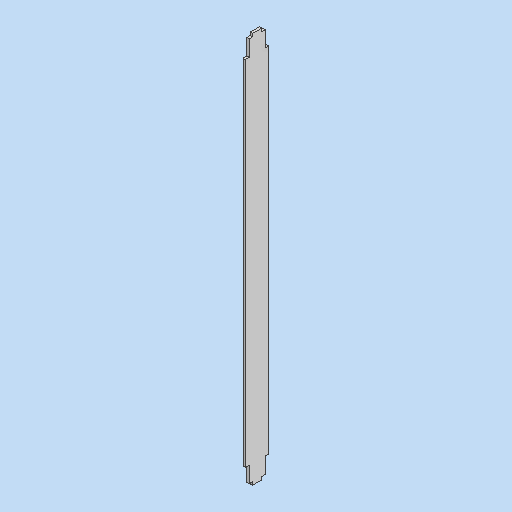
# Autodesk Inventor part: Acrly_Wand_1
Saved by Autodesk Inventor 2022 (Build 260153000, 153)
## iProperties
Created: 2021-12-15
Part Number: Acrly_Wand_1
Material: Generic
Document SubType Name: Modeling
Designer: Fabijansven
Density: 1 g/cm^3
Appearance: Default
Author: Fabijansven
Autodesk Inventor part; units mm, degrees
ref_plane "YZ Plane" through (0, 0, 0) normal (1, 0, 0) x (0, 1, 0)
ref_plane "XZ Plane" through (0, 0, 0) normal (0, 1, 0) x (-1, 0, 0)
ref_plane "XY Plane" through (0, 0, 0) normal (0, 0, 1) x (1, 0, 0)
sketch "Sketch1" plane through (0, 0, 0) normal (1, 0, 0) x (0, 1, 0)
  line L0 (0, 0) -> (822, 0)
  line L1 (822, 0) -> (822, -49.5)
  line L2 (822, -49.5) -> (0, -49.5)
  line L3 (0, -49.5) -> (0, 0)
  line L4 (822, 0) -> (815.75, 0)
  line L5 (815.75, 0) -> (815.75, -15)
  line L6 (815.75, -15) -> (822, -15)
  line L7 (822, -15) -> (822, 0)
  line L8 (822, 0) -> (782, 0)
  line L9 (782, 0) -> (782, -8)
  line L10 (782, -8) -> (822, -8)
  line L11 (822, -8) -> (822, 0)
  line L12 (856.5319, -24.75) -> (-65.1606, -24.75) construction
  line L13 (411, 165.682) -> (411, -1074.2454) construction
  line L14 (822, -49.5) -> (815.75, -49.5)
  line L15 (815.75, -49.5) -> (815.75, -34.5)
  line L16 (815.75, -34.5) -> (822, -34.5)
  line L17 (822, -34.5) -> (822, -49.5)
  line L18 (822, -49.5) -> (782, -49.5)
  line L19 (782, -49.5) -> (782, -41.5)
  line L20 (782, -41.5) -> (822, -41.5)
  line L21 (822, -41.5) -> (822, -49.5)
  line L22 (0, 0) -> (0, -49.5)
  line L23 (0, 0) -> (6.25, 0)
  line L24 (6.25, 0) -> (6.25, -15)
  line L25 (6.25, -15) -> (0, -15)
  line L26 (0, -15) -> (0, 0)
  line L27 (0, 0) -> (40, 0)
  line L28 (40, 0) -> (40, -8)
  line L29 (40, -8) -> (0, -8)
  line L30 (0, -8) -> (0, 0)
  line L31 (6.25, -34.5) -> (0, -34.5)
  line L32 (40, -41.5) -> (0, -41.5)
  line L33 (0, -49.5) -> (6.25, -49.5)
  line L34 (6.25, -49.5) -> (6.25, -34.5)
  line L35 (0, -34.5) -> (0, -49.5)
  line L36 (0, -49.5) -> (40, -49.5)
  line L37 (40, -49.5) -> (40, -41.5)
  line L38 (0, -41.5) -> (0, -49.5)
  point P0 (40, -49.5)
  point P1 (782, -49.5)
  point P2 (815.75, -41.5)
  point P3 (822, -34.5)
  point P4 (822, -15)
  point P5 (815.75, -8)
  point P6 (782, 0)
  point P7 (40, 0)
  point P8 (6.25, -8)
  point P9 (0, -15)
  point P10 (0, -34.5)
  point P11 (6.25, -41.5)
  dimension "d0" = 822
  dimension "d1" = 49.5
  dimension "d2" = 15
  dimension "d3" = 40
  dimension "d4" = 8
  dimension "d5" = 6.25
  dimension "d6" = 24.75
  dimension "d7" = 411
  constraints: 78 end point, 18 symmetric about line, 6 parallel, 4 horizontal, 3 perpendicular, 1 vertical
  measures "d0" distance of L1.end L2.end
  measures "d1" distance of L0.end L1.end
  measures "d2" distance of L4.end L5.end
  measures "d3" distance of L9.end L10.end
  measures "d4" distance of L8.end L9.end
  measures "d5" distance of L5.end L6.end
  measures "d6" distance between parallel lines of L0 L12
  measures "d7" distance between parallel lines of L3 L13
extrude "Extrusion1" add sketch "Sketch1" along normal blind 5 contours L0 L9 L10 L5 L6 L1 L16 L15 L20 L19 L2 L37 L32 L34 L31 L3 L25 L24 L29 L28
equation "\"d6\" = 0.5 * d1"
equation "\"d7\" = 0.5 * d0"
body "Solid1"
